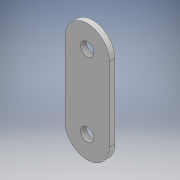
# Autodesk Inventor part: LRF Clamp
Saved by Autodesk Inventor 2018 (Build 220112000, 112)
## iProperties
Created: 2018-09-27
Part Number: LRF Clamp
Material: Generic
Document SubType Name: Modeling
Designer: matth
Density: 1 g/cm^3
Appearance: Default
Author: matth
Autodesk Inventor part; units mm, degrees
ref_plane "YZ Plane" through (0, 0, 0) normal (1, 0, 0) x (0, 1, 0)
ref_plane "XZ Plane" through (0, 0, 0) normal (0, 1, 0) x (-1, 0, 0)
ref_plane "XY Plane" through (0, 0, 0) normal (0, 0, 1) x (1, 0, 0)
sketch "Sketch1" plane through (0, 0, 0) normal (0, 1, 0) x (-1, 0, 0)
  line L0 (0, 0) -> (0, -20)
  circle A0 centre (0, 0) radius 1.75
  circle A1 centre (0, -20) radius 1.75
  line L1 (0, 0) -> (0, -20) construction
  line L2 (-6, 0) -> (-6, -20)
  line L3 (6, -20) -> (6, 0)
  arc A2 (6, 0) -> (-6, 0) centre (0, 0) ccw
  arc A3 (-6, -20) -> (6, -20) centre (0, -20) ccw
  point P0 (0, -10)
  dimension "d0" = 20
  dimension "d1" = 3.5
  dimension "d2" = 3.5
  dimension "d3" = 12
  constraints: 10 end point, 4 centre point, 4 point on circle, 4 tangent, 2 coincident, 2 vertical, 1 midpoint, 1 parallel
  measures "d0" distance of L0.start L0.end
  measures "d1" diameter of A0
  measures "d2" diameter of A1
  measures "d3" diameter of A3
extrude "Extrusion1" add sketch "Sketch1" along normal blind 1.5
body "Solid1"
